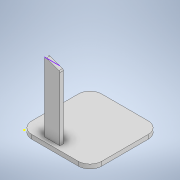
# Autodesk Inventor part: SmartWatch_Base
Saved by Autodesk Inventor 2020.1 (Build 241239000, 239)
## iProperties
Created: 2020-02-16
Part Number: SmartWatch_Base
Material: Generic
Document SubType Name: Modeling
Designer: super
Density: 1 g/cm^3
Appearance: Default
Author: super
Autodesk Inventor part; units mm, degrees
ref_plane "YZ Plane" through (0, 0, 0) normal (1, 0, 0) x (0, 1, 0)
ref_plane "XZ Plane" through (0, 0, 0) normal (0, 1, 0) x (-1, 0, 0)
ref_plane "XY Plane" through (0, 0, 0) normal (0, 0, 1) x (1, 0, 0)
sketch "Sketch1" plane through (0, 0, 0) normal (0, 1, 0) x (-1, 0, 0)
  line L0 (0, 0) -> (-100, 0)
  line L1 (-100, 0) -> (-100, -100)
  line L2 (-100, -100) -> (0, -100)
  line L3 (0, -100) -> (0, 0)
  dimension "d0" = 100
  dimension "d1" = 100
  constraints: 8 end point, 2 parallel, 1 horizontal, 1 perpendicular
  measures "d0" distance of L2.end L1.end
  measures "d1" distance of L1.end L0.end
extrude "Extrusion1" add sketch "Sketch1" along normal blind 6
fillet "Fillet1" radius 16.75 4 edges at (100, 3, 0) (100, 3, -100) (0, 3, 0) (0, 3, -100)
sketch "Sketch2" plane through (0, 6, 0) normal (0, 1, 0) x (1, 0, 0)
  line L0 (16.75, 0) -> (83.25, 0) projected
  line L1 (40, 6) -> (51, 6)
  line L2 (51, 6) -> (51, 11)
  line L3 (51, 11) -> (29, 11)
  line L4 (29, 11) -> (29, 6)
  line L5 (29, 6) -> (40, 6)
  point P0 (0, 0)
  constraints: 10 end point, 4 perpendicular, 1 point on line
extrude "Extrusion2" add sketch "Sketch2" along normal blind 100
sketch "Sketch3" plane through (29, 6, -6) normal (0, 0, 1) x (1, 0, 0)
  line L0 (0, 100) -> (22, 100) projected
  line L1 (0, 100) -> (22, 91.9927)
  line L2 (22, 0) -> (22, 100) projected
  line L3 (0, 100) -> (23.4119, 100) construction
  line L4 (22, 91.9927) -> (22, 100)
  line L5 (22, 100) -> (0, 100)
  point P0 (-29, -6)
  dimension "d12" = 20
  constraints: 8 end point, 1 collinear, 1 equal length, 1 horizontal, 1 perpendicular, 1 point on line
  measures "d12" angle of L1 L3
extrude "Extrusion3" cut sketch "Sketch3" against normal blind 10
fillet "Fillet2" radius 2 2 edges at (29, 106, -8.5) (51, 97.9927, -8.5)
sketch "Sketch4" plane through (51, 6, -11) normal (0, 0, -1) x (-1, 0, 0)
  point P0 (51, -6)
sketch "Sketch5" plane through (29, 6, -6) normal (0, 0, 1) x (1, 0, 0)
  line L0 (0, 99.0231) -> (22, 99.0231)
  point P0 (-29, -6)
  constraints: 2 end point, 1 horizontal
body "Solid1"
